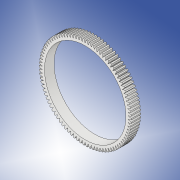
# Autodesk Inventor part: Flexspline
Saved by Autodesk Inventor 2017 (Build 210142000, 142)
## iProperties
Created: 2017-07-11
Part Number: Flexspline
Material: ABS Plastic
Document SubType Name: Modeling
Designer: zallen
Density: 1.06 g/cm^3
Appearance: CR White
Author: zallen
Autodesk Inventor part; units mm, degrees
ref_plane "YZ Plane" through (0, 0, 0) normal (1, 0, 0) x (0, 1, 0)
ref_plane "XZ Plane" through (0, 0, 0) normal (0, 1, 0) x (-1, 0, 0)
ref_plane "XY Plane" through (0, 0, 0) normal (0, 0, 1) x (1, 0, 0)
sketch "Sketch1" plane through (0, 0, 0) normal (0, 0, 1) x (1, 0, 0)
  circle A0 centre (0, 0) radius 45
  circle A1 centre (0, 0) radius 48 construction
  line L0 (0, 0) -> (52.2063, 0) construction
  arc A2 (47.9962, 0.6) -> (44.9782, 1.4) centre (42.6647, -13.4205) ccw
  arc A3 (47.9962, -0.6) -> (47.9962, 0.6) centre (28.0053, 0) ccw
  arc A4 (44.9782, -1.4) -> (47.9962, -0.6) centre (42.6647, 13.4205) ccw
  arc A5 (44.9782, -1.4) -> (44.9782, 1.4) centre (0, 0) ccw
  arc A6 (47.8375, 3.9466) -> (44.771, 4.5341) centre (43.497, -10.4117) ccw
  arc A7 (44.9663, 1.7409) -> (47.9212, 2.7495) centre (41.6246, 16.364) ccw
  arc A8 (47.9212, 2.7495) -> (47.8375, 3.9466) centre (27.937, 1.9535) ccw
  circle A9 centre (0, 0) radius 45
  arc A10 (44.9663, 1.7409) -> (44.771, 4.5341) centre (0, 0) ccw
  arc A11 (47.4456, 7.2739) -> (44.3456, 7.6461) centre (44.1173, -7.3521) ccw
  arc A12 (44.7353, 4.8734) -> (47.6127, 6.0856) centre (40.3818, 19.2277) ccw
  arc A13 (47.6127, 6.0856) -> (47.4456, 7.2739) centre (27.7327, 3.8976) ccw
  circle A14 centre (0, 0) radius 45
  arc A15 (44.7353, 4.8734) -> (44.3456, 7.6461) centre (0, 0) ccw
  arc A16 (46.8227, 10.5659) -> (43.7043, 10.7209) centre (44.5227, -4.2568) ccw
  arc A17 (44.2864, 7.9821) -> (47.0722, 9.3921) centre (38.9421, 21.9977) ccw
  arc A18 (47.0722, 9.3921) -> (46.8227, 10.5659) centre (27.3933, 5.8226) ccw
  circle A19 centre (0, 0) radius 45
  arc A20 (44.2864, 7.9821) -> (43.7043, 10.7209) centre (0, 0) ccw
  arc A21 (45.9716, 13.8063) -> (42.8499, 13.7434) centre (44.7112, -1.1406) ccw
  arc A22 (43.6217, 11.0519) -> (46.3023, 12.6528) centre (37.3128, 24.6606) ccw
  arc A23 (46.3023, 12.6528) -> (45.9716, 13.8063) centre (26.9204, 7.7193) ccw
  circle A24 centre (0, 0) radius 45
  arc A25 (43.6217, 11.0519) -> (42.8499, 13.7434) centre (0, 0) ccw
  arc A26 (44.8965, 16.9795) -> (41.7869, 16.699) centre (44.6818, 1.981) ccw
  arc A27 (42.7445, 14.0679) -> (45.3069, 15.8519) centre (35.5017, 27.2034) ccw
  arc A28 (45.3069, 15.8519) -> (44.8965, 16.9795) centre (26.3163, 9.5784) ccw
  circle A29 centre (0, 0) radius 45
  arc A30 (42.7445, 14.0679) -> (41.7869, 16.699) centre (0, 0) ccw
  arc A31 (43.6027, 20.07) -> (40.5202, 19.5733) centre (44.4348, 5.0931) ccw
  arc A32 (41.6591, 17.0153) -> (44.0908, 18.9737) centre (33.5176, 29.6136) ccw
  arc A33 (44.0908, 18.9737) -> (43.6027, 20.07) centre (25.5841, 11.3908) ccw
  circle A34 centre (0, 0) radius 45
  arc A35 (41.6591, 17.0153) -> (40.5202, 19.5733) centre (0, 0) ccw
  arc A36 (42.0965, 23.0626) -> (39.0561, 22.3521) centre (43.9713, 8.1803) ccw
  arc A37 (40.3707, 19.8799) -> (42.6599, 22.0031) centre (31.3702, 31.8795) ccw
  arc A38 (42.6599, 22.0031) -> (42.0965, 23.0626) centre (24.7272, 13.1477) ccw
  circle A39 centre (0, 0) radius 45
  arc A40 (40.3707, 19.8799) -> (39.0561, 22.3521) centre (0, 0) ccw
  arc A41 (40.3852, 25.943) -> (37.4018, 25.0221) centre (43.2935, 11.2276) ccw
  arc A42 (38.8856, 22.6476) -> (41.0211, 24.9253) centre (29.07, 33.9901) ccw
  arc A43 (41.0211, 24.9253) -> (40.3852, 25.943) centre (23.7498, 14.8405) ccw
  circle A44 centre (0, 0) radius 45
  arc A45 (38.8856, 22.6476) -> (37.4018, 25.0221) centre (0, 0) ccw
  arc A46 (38.4771, 28.6969) -> (35.5652, 27.5702) centre (42.4049, 14.2203) ccw
  arc A47 (37.211, 25.3049) -> (39.1825, 27.7261) centre (26.6281, 35.9351) ccw
  arc A48 (39.1825, 27.7261) -> (38.4771, 28.6969) centre (22.6567, 16.4611) ccw
  circle A49 centre (0, 0) radius 45
  arc A50 (37.211, 25.3049) -> (35.5652, 27.5702) centre (0, 0) ccw
  arc A51 (36.3816, 31.311) -> (33.5554, 29.9839) centre (41.3096, 17.1437) ccw
  arc A52 (35.3552, 27.839) -> (37.1529, 30.3918) centre (24.0565, 37.7051) ccw
  arc A53 (37.1529, 30.3918) -> (36.3816, 31.311) centre (21.4533, 18.0014) ccw
  circle A54 centre (0, 0) radius 45
  arc A55 (35.3552, 27.839) -> (33.5554, 29.9839) centre (0, 0) ccw
  arc A56 (34.1088, 33.7726) -> (31.3821, 32.2516) centre (40.0131, 19.9835) ccw
  arc A57 (33.3271, 30.2374) -> (34.9424, 32.9094) centre (21.3678, 39.2913) ccw
  arc A58 (34.9424, 32.9094) -> (34.1088, 33.7726) centre (20.1453, 19.4541) ccw
  circle A59 centre (0, 0) radius 45
  arc A60 (33.3271, 30.2374) -> (31.3821, 32.2516) centre (0, 0) ccw
  arc A61 (31.6699, 36.0696) -> (29.0559, 34.3621) centre (38.5217, 22.726) ccw
  arc A62 (31.1367, 32.4885) -> (32.5616, 35.2667) centre (18.5749, 40.6862) ccw
  arc A63 (32.5616, 35.2667) -> (31.6699, 36.0696) centre (18.7392, 20.812) ccw
  circle A64 centre (0, 0) radius 45
  arc A65 (31.1367, 32.4885) -> (29.0559, 34.3621) centre (0, 0) ccw
  arc A66 (29.0766, 38.191) -> (26.5881, 36.3052) centre (36.8425, 25.3578) ccw
  arc A67 (28.7946, 34.5814) -> (30.0222, 37.4522) centre (15.6915, 41.8828) ccw
  arc A68 (30.0222, 37.4522) -> (29.0766, 38.191) centre (17.2418, 22.0684) ccw
  circle A69 centre (0, 0) radius 45
  arc A70 (28.7946, 34.5814) -> (26.5881, 36.3052) centre (0, 0) ccw
  arc A71 (26.3417, 40.1262) -> (23.9908, 38.0715) centre (34.9839, 27.866) ccw
  arc A72 (26.3122, 36.5058) -> (27.3366, 39.4552) centre (12.7317, 42.8753) ccw
  arc A73 (27.3366, 39.4552) -> (26.3417, 40.1262) centre (15.6603, 23.2174) ccw
  circle A74 centre (0, 0) radius 45
  arc A75 (26.3122, 36.5058) -> (23.9908, 38.0715) centre (0, 0) ccw
  arc A76 (23.4785, 41.866) -> (21.2767, 39.6523) centre (32.9549, 30.2385) ccw
  arc A77 (23.7015, 38.2523) -> (24.5177, 41.266) centre (9.7099, 43.659) ccw
  arc A78 (24.5177, 41.266) -> (23.4785, 41.866) centre (14.0026, 24.2533) ccw
  circle A79 centre (0, 0) radius 45
  arc A80 (23.7015, 38.2523) -> (21.2767, 39.6523) centre (0, 0) ccw
  arc A81 (20.5009, 43.4018) -> (18.4588, 41.0399) centre (30.7653, 32.4636) ccw
  arc A82 (20.9755, 39.8124) -> (21.5794, 42.8757) centre (6.6407, 44.23) ccw
  arc A83 (21.5794, 42.8757) -> (20.5009, 43.4018) centre (12.2767, 25.171) ccw
  circle A84 centre (0, 0) radius 45
  arc A85 (20.9755, 39.8124) -> (18.4588, 41.0399) centre (0, 0) ccw
  arc A86 (17.4234, 44.7261) -> (15.5511, 42.2275) centre (28.4258, 34.5306) ccw
  arc A87 (18.1472, 41.1786) -> (18.536, 44.2766) centre (3.5392, 44.5855) ccw
  arc A88 (18.536, 44.2766) -> (17.4234, 44.7261) centre (10.491, 25.966) ccw
  circle A89 centre (0, 0) radius 45
  arc A90 (18.1472, 41.1786) -> (15.5511, 42.2275) centre (0, 0) ccw
  arc A91 (14.261, 45.8326) -> (12.5676, 43.2095) centre (25.9478, 36.4294) ccw
  arc A92 (15.2305, 42.3442) -> (15.4023, 45.4617) centre (0.4205, 44.7237) ccw
  arc A93 (15.4023, 45.4617) -> (14.261, 45.8326) centre (8.6541, 26.6346) ccw
  circle A94 centre (0, 0) radius 45
  arc A95 (15.2305, 42.3442) -> (12.5676, 43.2095) centre (0, 0) ccw
  arc A96 (11.0292, 46.7157) -> (9.5228, 43.9809) centre (23.3434, 38.1507) ccw
  arc A97 (12.2396, 43.3035) -> (12.1935, 46.4254) centre (-2.7003, 44.6441) ccw
  arc A98 (12.1935, 46.4254) -> (11.0292, 46.7157) centre (6.7751, 27.1734) ccw
  circle A99 centre (0, 0) radius 45
  arc A100 (12.2396, 43.3035) -> (9.5228, 43.9809) centre (0, 0) ccw
  arc A101 (7.7436, 47.3713) -> (6.4317, 44.538) centre (20.6253, 39.6861) ccw
  arc A102 (9.1891, 44.0518) -> (8.9253, 47.1629) centre (-5.808, 44.347) ccw
  arc A103 (8.9253, 47.1629) -> (7.7436, 47.3713) centre (4.8631, 27.5798) ccw
  circle A104 centre (0, 0) radius 45
  arc A105 (9.1891, 44.0518) -> (6.4317, 44.538) centre (0, 0) ccw
  arc A106 (4.4203, 47.796) -> (3.3092, 44.8782) centre (17.8067, 41.0282) ccw
  arc A107 (6.0938, 44.5855) -> (5.6137, 47.6706) centre (-8.8873, 43.8338) ccw
  arc A108 (5.6137, 47.6706) -> (4.4203, 47.796) centre (2.9273, 27.8518) ccw
  circle A109 centre (0, 0) radius 45
  arc A110 (6.0938, 44.5855) -> (3.3092, 44.8782) centre (0, 0) ccw
  arc A111 (1.0754, 47.988) -> (0.1706, 44.9997) centre (14.9013, 42.1704) ccw
  arc A112 (2.9689, 44.902) -> (2.2747, 47.9461) centre (-11.9234, 43.1071) ccw
  arc A113 (2.2747, 47.9461) -> (1.0754, 47.988) centre (0.9774, 27.9882) ccw
  circle A114 centre (0, 0) radius 45
  arc A115 (2.9689, 44.902) -> (0.1706, 44.9997) centre (0, 0) ccw
  arc A116 (-2.2747, 47.9461) -> (-2.9689, 44.902) centre (11.9234, 43.1071) ccw
  arc A117 (-0.1706, 44.9997) -> (-1.0754, 47.988) centre (-14.9013, 42.1704) ccw
  arc A118 (-1.0754, 47.988) -> (-2.2747, 47.9461) centre (-0.9774, 27.9882) ccw
  circle A119 centre (0, 0) radius 45
  arc A120 (-0.1706, 44.9997) -> (-2.9689, 44.902) centre (0, 0) ccw
  arc A121 (-5.6137, 47.6706) -> (-6.0938, 44.5855) centre (8.8873, 43.8338) ccw
  arc A122 (-3.3092, 44.8782) -> (-4.4203, 47.796) centre (-17.8067, 41.0282) ccw
  arc A123 (-4.4203, 47.796) -> (-5.6137, 47.6706) centre (-2.9273, 27.8518) ccw
  circle A124 centre (0, 0) radius 45
  arc A125 (-3.3092, 44.8782) -> (-6.0938, 44.5855) centre (0, 0) ccw
  arc A126 (-8.9253, 47.1629) -> (-9.1891, 44.0518) centre (5.808, 44.347) ccw
  arc A127 (-6.4317, 44.538) -> (-7.7436, 47.3713) centre (-20.6253, 39.6861) ccw
  arc A128 (-7.7436, 47.3713) -> (-8.9253, 47.1629) centre (-4.8631, 27.5798) ccw
  circle A129 centre (0, 0) radius 45
  arc A130 (-6.4317, 44.538) -> (-9.1891, 44.0518) centre (0, 0) ccw
  arc A131 (-12.1935, 46.4254) -> (-12.2396, 43.3035) centre (2.7003, 44.6441) ccw
  arc A132 (-9.5228, 43.9809) -> (-11.0292, 46.7157) centre (-23.3434, 38.1507) ccw
  arc A133 (-11.0292, 46.7157) -> (-12.1935, 46.4254) centre (-6.7751, 27.1734) ccw
  circle A134 centre (0, 0) radius 45
  arc A135 (-9.5228, 43.9809) -> (-12.2396, 43.3035) centre (0, 0) ccw
  arc A136 (-15.4023, 45.4617) -> (-15.2305, 42.3442) centre (-0.4205, 44.7237) ccw
  arc A137 (-12.5676, 43.2095) -> (-14.261, 45.8326) centre (-25.9478, 36.4294) ccw
  arc A138 (-14.261, 45.8326) -> (-15.4023, 45.4617) centre (-8.6541, 26.6346) ccw
  circle A139 centre (0, 0) radius 45
  arc A140 (-12.5676, 43.2095) -> (-15.2305, 42.3442) centre (0, 0) ccw
  arc A141 (-18.536, 44.2766) -> (-18.1472, 41.1786) centre (-3.5392, 44.5855) ccw
  arc A142 (-15.5511, 42.2275) -> (-17.4234, 44.7261) centre (-28.4258, 34.5306) ccw
  arc A143 (-17.4234, 44.7261) -> (-18.536, 44.2766) centre (-10.491, 25.966) ccw
  circle A144 centre (0, 0) radius 45
  arc A145 (-15.5511, 42.2275) -> (-18.1472, 41.1786) centre (0, 0) ccw
  arc A146 (-21.5794, 42.8757) -> (-20.9755, 39.8124) centre (-6.6407, 44.23) ccw
  arc A147 (-18.4588, 41.0399) -> (-20.5009, 43.4018) centre (-30.7653, 32.4636) ccw
  arc A148 (-20.5009, 43.4018) -> (-21.5794, 42.8757) centre (-12.2767, 25.171) ccw
  circle A149 centre (0, 0) radius 45
  arc A150 (-18.4588, 41.0399) -> (-20.9755, 39.8124) centre (0, 0) ccw
  arc A151 (-24.5177, 41.266) -> (-23.7015, 38.2523) centre (-9.7099, 43.659) ccw
  arc A152 (-21.2767, 39.6523) -> (-23.4785, 41.866) centre (-32.9549, 30.2385) ccw
  arc A153 (-23.4785, 41.866) -> (-24.5177, 41.266) centre (-14.0026, 24.2533) ccw
  circle A154 centre (0, 0) radius 45
  arc A155 (-21.2767, 39.6523) -> (-23.7015, 38.2523) centre (0, 0) ccw
  arc A156 (-27.3366, 39.4552) -> (-26.3122, 36.5058) centre (-12.7317, 42.8753) ccw
  arc A157 (-23.9908, 38.0715) -> (-26.3417, 40.1262) centre (-34.9839, 27.866) ccw
  arc A158 (-26.3417, 40.1262) -> (-27.3366, 39.4552) centre (-15.6603, 23.2174) ccw
  circle A159 centre (0, 0) radius 45
  arc A160 (-23.9908, 38.0715) -> (-26.3122, 36.5058) centre (0, 0) ccw
  arc A161 (-30.0222, 37.4522) -> (-28.7946, 34.5814) centre (-15.6915, 41.8828) ccw
  arc A162 (-26.5881, 36.3052) -> (-29.0766, 38.191) centre (-36.8425, 25.3578) ccw
  arc A163 (-29.0766, 38.191) -> (-30.0222, 37.4522) centre (-17.2418, 22.0684) ccw
  circle A164 centre (0, 0) radius 45
  arc A165 (-26.5881, 36.3052) -> (-28.7946, 34.5814) centre (0, 0) ccw
  arc A166 (-32.5616, 35.2667) -> (-31.1367, 32.4885) centre (-18.5749, 40.6862) ccw
  arc A167 (-29.0559, 34.3621) -> (-31.6699, 36.0696) centre (-38.5217, 22.726) ccw
  arc A168 (-31.6699, 36.0696) -> (-32.5616, 35.2667) centre (-18.7392, 20.812) ccw
  circle A169 centre (0, 0) radius 45
  arc A170 (-29.0559, 34.3621) -> (-31.1367, 32.4885) centre (0, 0) ccw
  arc A171 (-34.9424, 32.9094) -> (-33.3271, 30.2374) centre (-21.3678, 39.2913) ccw
  arc A172 (-31.3821, 32.2516) -> (-34.1088, 33.7726) centre (-40.0131, 19.9835) ccw
  arc A173 (-34.1088, 33.7726) -> (-34.9424, 32.9094) centre (-20.1453, 19.4541) ccw
  circle A174 centre (0, 0) radius 45
  arc A175 (-31.3821, 32.2516) -> (-33.3271, 30.2374) centre (0, 0) ccw
  arc A176 (-37.1529, 30.3918) -> (-35.3552, 27.839) centre (-24.0565, 37.7051) ccw
  arc A177 (-33.5554, 29.9839) -> (-36.3816, 31.311) centre (-41.3096, 17.1437) ccw
  arc A178 (-36.3816, 31.311) -> (-37.1529, 30.3918) centre (-21.4533, 18.0014) ccw
  circle A179 centre (0, 0) radius 45
  arc A180 (-33.5554, 29.9839) -> (-35.3552, 27.839) centre (0, 0) ccw
  arc A181 (-39.1825, 27.7261) -> (-37.211, 25.3049) centre (-26.6281, 35.9351) ccw
  arc A182 (-35.5652, 27.5702) -> (-38.4771, 28.6969) centre (-42.4049, 14.2203) ccw
  arc A183 (-38.4771, 28.6969) -> (-39.1825, 27.7261) centre (-22.6567, 16.4611) ccw
  circle A184 centre (0, 0) radius 45
  arc A185 (-35.5652, 27.5702) -> (-37.211, 25.3049) centre (0, 0) ccw
  arc A186 (-41.0211, 24.9253) -> (-38.8856, 22.6476) centre (-29.07, 33.9901) ccw
  arc A187 (-37.4018, 25.0221) -> (-40.3852, 25.943) centre (-43.2935, 11.2276) ccw
  arc A188 (-40.3852, 25.943) -> (-41.0211, 24.9253) centre (-23.7498, 14.8405) ccw
  circle A189 centre (0, 0) radius 45
  arc A190 (-37.4018, 25.0221) -> (-38.8856, 22.6476) centre (0, 0) ccw
  arc A191 (-42.6599, 22.0031) -> (-40.3707, 19.8799) centre (-31.3702, 31.8795) ccw
  arc A192 (-39.0561, 22.3521) -> (-42.0965, 23.0626) centre (-43.9713, 8.1803) ccw
  arc A193 (-42.0965, 23.0626) -> (-42.6599, 22.0031) centre (-24.7272, 13.1477) ccw
  circle A194 centre (0, 0) radius 45
  arc A195 (-39.0561, 22.3521) -> (-40.3707, 19.8799) centre (0, 0) ccw
  arc A196 (-44.0908, 18.9737) -> (-41.6591, 17.0153) centre (-33.5176, 29.6136) ccw
  arc A197 (-40.5202, 19.5733) -> (-43.6027, 20.07) centre (-44.4348, 5.0931) ccw
  arc A198 (-43.6027, 20.07) -> (-44.0908, 18.9737) centre (-25.5841, 11.3908) ccw
  circle A199 centre (0, 0) radius 45
  arc A200 (-40.5202, 19.5733) -> (-41.6591, 17.0153) centre (0, 0) ccw
  arc A201 (-45.3069, 15.8519) -> (-42.7445, 14.0679) centre (-35.5017, 27.2034) ccw
  arc A202 (-41.7869, 16.699) -> (-44.8965, 16.9795) centre (-44.6818, 1.981) ccw
  arc A203 (-44.8965, 16.9795) -> (-45.3069, 15.8519) centre (-26.3163, 9.5784) ccw
  circle A204 centre (0, 0) radius 45
  arc A205 (-41.7869, 16.699) -> (-42.7445, 14.0679) centre (0, 0) ccw
  arc A206 (-46.3023, 12.6528) -> (-43.6217, 11.0519) centre (-37.3128, 24.6606) ccw
  arc A207 (-42.8499, 13.7434) -> (-45.9716, 13.8063) centre (-44.7112, -1.1406) ccw
  arc A208 (-45.9716, 13.8063) -> (-46.3023, 12.6528) centre (-26.9204, 7.7193) ccw
  circle A209 centre (0, 0) radius 45
  arc A210 (-42.8499, 13.7434) -> (-43.6217, 11.0519) centre (0, 0) ccw
  arc A211 (-47.0722, 9.3921) -> (-44.2864, 7.9821) centre (-38.9421, 21.9977) ccw
  arc A212 (-43.7043, 10.7209) -> (-46.8227, 10.5659) centre (-44.5227, -4.2568) ccw
  arc A213 (-46.8227, 10.5659) -> (-47.0722, 9.3921) centre (-27.3933, 5.8226) ccw
  circle A214 centre (0, 0) radius 45
  arc A215 (-43.7043, 10.7209) -> (-44.2864, 7.9821) centre (0, 0) ccw
  arc A216 (-47.6127, 6.0856) -> (-44.7353, 4.8734) centre (-40.3818, 19.2277) ccw
  arc A217 (-44.3456, 7.6461) -> (-47.4456, 7.2739) centre (-44.1173, -7.3521) ccw
  arc A218 (-47.4456, 7.2739) -> (-47.6127, 6.0856) centre (-27.7327, 3.8976) ccw
  circle A219 centre (0, 0) radius 45
  arc A220 (-44.3456, 7.6461) -> (-44.7353, 4.8734) centre (0, 0) ccw
  arc A221 (-47.9212, 2.7495) -> (-44.9663, 1.7409) centre (-41.6246, 16.364) ccw
  arc A222 (-44.771, 4.5341) -> (-47.8375, 3.9466) centre (-43.497, -10.4117) ccw
  arc A223 (-47.8375, 3.9466) -> (-47.9212, 2.7495) centre (-27.937, 1.9535) ccw
  circle A224 centre (0, 0) radius 45
  arc A225 (-44.771, 4.5341) -> (-44.9663, 1.7409) centre (0, 0) ccw
  arc A226 (-47.9962, -0.6) -> (-44.9782, -1.4) centre (-42.6647, 13.4205) ccw
  arc A227 (-44.9782, 1.4) -> (-47.9962, 0.6) centre (-42.6647, -13.4205) ccw
  arc A228 (-47.9962, 0.6) -> (-47.9962, -0.6) centre (-28.0053, 0) ccw
  circle A229 centre (0, 0) radius 45
  arc A230 (-44.9782, 1.4) -> (-44.9782, -1.4) centre (0, 0) ccw
  arc A231 (-47.8375, -3.9466) -> (-44.771, -4.5341) centre (-43.497, 10.4117) ccw
  arc A232 (-44.9663, -1.7409) -> (-47.9212, -2.7495) centre (-41.6246, -16.364) ccw
  arc A233 (-47.9212, -2.7495) -> (-47.8375, -3.9466) centre (-27.937, -1.9535) ccw
  circle A234 centre (0, 0) radius 45
  arc A235 (-44.9663, -1.7409) -> (-44.771, -4.5341) centre (0, 0) ccw
  arc A236 (-47.4456, -7.2739) -> (-44.3456, -7.6461) centre (-44.1173, 7.3521) ccw
  arc A237 (-44.7353, -4.8734) -> (-47.6127, -6.0856) centre (-40.3818, -19.2277) ccw
  arc A238 (-47.6127, -6.0856) -> (-47.4456, -7.2739) centre (-27.7327, -3.8976) ccw
  circle A239 centre (0, 0) radius 45
  arc A240 (-44.7353, -4.8734) -> (-44.3456, -7.6461) centre (0, 0) ccw
  arc A241 (-46.8227, -10.5659) -> (-43.7043, -10.7209) centre (-44.5227, 4.2568) ccw
  arc A242 (-44.2864, -7.9821) -> (-47.0722, -9.3921) centre (-38.9421, -21.9977) ccw
  arc A243 (-47.0722, -9.3921) -> (-46.8227, -10.5659) centre (-27.3933, -5.8226) ccw
  circle A244 centre (0, 0) radius 45
  arc A245 (-44.2864, -7.9821) -> (-43.7043, -10.7209) centre (0, 0) ccw
  arc A246 (-45.9716, -13.8063) -> (-42.8499, -13.7434) centre (-44.7112, 1.1406) ccw
  arc A247 (-43.6217, -11.0519) -> (-46.3023, -12.6528) centre (-37.3128, -24.6606) ccw
  arc A248 (-46.3023, -12.6528) -> (-45.9716, -13.8063) centre (-26.9204, -7.7193) ccw
  circle A249 centre (0, 0) radius 45
  arc A250 (-43.6217, -11.0519) -> (-42.8499, -13.7434) centre (0, 0) ccw
  arc A251 (-44.8965, -16.9795) -> (-41.7869, -16.699) centre (-44.6818, -1.981) ccw
  arc A252 (-42.7445, -14.0679) -> (-45.3069, -15.8519) centre (-35.5017, -27.2034) ccw
  arc A253 (-45.3069, -15.8519) -> (-44.8965, -16.9795) centre (-26.3163, -9.5784) ccw
  circle A254 centre (0, 0) radius 45
  arc A255 (-42.7445, -14.0679) -> (-41.7869, -16.699) centre (0, 0) ccw
  arc A256 (-43.6027, -20.07) -> (-40.5202, -19.5733) centre (-44.4348, -5.0931) ccw
  arc A257 (-41.6591, -17.0153) -> (-44.0908, -18.9737) centre (-33.5176, -29.6136) ccw
  arc A258 (-44.0908, -18.9737) -> (-43.6027, -20.07) centre (-25.5841, -11.3908) ccw
  circle A259 centre (0, 0) radius 45
  arc A260 (-41.6591, -17.0153) -> (-40.5202, -19.5733) centre (0, 0) ccw
  arc A261 (-42.0965, -23.0626) -> (-39.0561, -22.3521) centre (-43.9713, -8.1803) ccw
  arc A262 (-40.3707, -19.8799) -> (-42.6599, -22.0031) centre (-31.3702, -31.8795) ccw
  arc A263 (-42.6599, -22.0031) -> (-42.0965, -23.0626) centre (-24.7272, -13.1477) ccw
  circle A264 centre (0, 0) radius 45
  arc A265 (-40.3707, -19.8799) -> (-39.0561, -22.3521) centre (0, 0) ccw
  arc A266 (-40.3852, -25.943) -> (-37.4018, -25.0221) centre (-43.2935, -11.2276) ccw
  arc A267 (-38.8856, -22.6476) -> (-41.0211, -24.9253) centre (-29.07, -33.9901) ccw
  arc A268 (-41.0211, -24.9253) -> (-40.3852, -25.943) centre (-23.7498, -14.8405) ccw
  circle A269 centre (0, 0) radius 45
  arc A270 (-38.8856, -22.6476) -> (-37.4018, -25.0221) centre (0, 0) ccw
  arc A271 (-38.4771, -28.6969) -> (-35.5652, -27.5702) centre (-42.4049, -14.2203) ccw
  arc A272 (-37.211, -25.3049) -> (-39.1825, -27.7261) centre (-26.6281, -35.9351) ccw
  arc A273 (-39.1825, -27.7261) -> (-38.4771, -28.6969) centre (-22.6567, -16.4611) ccw
  circle A274 centre (0, 0) radius 45
  arc A275 (-37.211, -25.3049) -> (-35.5652, -27.5702) centre (0, 0) ccw
  arc A276 (-36.3816, -31.311) -> (-33.5554, -29.9839) centre (-41.3096, -17.1437) ccw
  arc A277 (-35.3552, -27.839) -> (-37.1529, -30.3918) centre (-24.0565, -37.7051) ccw
  arc A278 (-37.1529, -30.3918) -> (-36.3816, -31.311) centre (-21.4533, -18.0014) ccw
  circle A279 centre (0, 0) radius 45
  arc A280 (-35.3552, -27.839) -> (-33.5554, -29.9839) centre (0, 0) ccw
  arc A281 (-34.1088, -33.7726) -> (-31.3821, -32.2516) centre (-40.0131, -19.9835) ccw
  arc A282 (-33.3271, -30.2374) -> (-34.9424, -32.9094) centre (-21.3678, -39.2913) ccw
  arc A283 (-34.9424, -32.9094) -> (-34.1088, -33.7726) centre (-20.1453, -19.4541) ccw
  circle A284 centre (0, 0) radius 45
  arc A285 (-33.3271, -30.2374) -> (-31.3821, -32.2516) centre (0, 0) ccw
  arc A286 (-31.6699, -36.0696) -> (-29.0559, -34.3621) centre (-38.5217, -22.726) ccw
  arc A287 (-31.1367, -32.4885) -> (-32.5616, -35.2667) centre (-18.5749, -40.6862) ccw
  arc A288 (-32.5616, -35.2667) -> (-31.6699, -36.0696) centre (-18.7392, -20.812) ccw
  circle A289 centre (0, 0) radius 45
  arc A290 (-31.1367, -32.4885) -> (-29.0559, -34.3621) centre (0, 0) ccw
  arc A291 (-29.0766, -38.191) -> (-26.5881, -36.3052) centre (-36.8425, -25.3578) ccw
  arc A292 (-28.7946, -34.5814) -> (-30.0222, -37.4522) centre (-15.6915, -41.8828) ccw
  arc A293 (-30.0222, -37.4522) -> (-29.0766, -38.191) centre (-17.2418, -22.0684) ccw
  circle A294 centre (0, 0) radius 45
  arc A295 (-28.7946, -34.5814) -> (-26.5881, -36.3052) centre (0, 0) ccw
  arc A296 (-26.3417, -40.1262) -> (-23.9908, -38.0715) centre (-34.9839, -27.866) ccw
  arc A297 (-26.3122, -36.5058) -> (-27.3366, -39.4552) centre (-12.7317, -42.8753) ccw
  arc A298 (-27.3366, -39.4552) -> (-26.3417, -40.1262) centre (-15.6603, -23.2174) ccw
  circle A299 centre (0, 0) radius 45
  arc A300 (-26.3122, -36.5058) -> (-23.9908, -38.0715) centre (0, 0) ccw
  arc A301 (-23.4785, -41.866) -> (-21.2767, -39.6523) centre (-32.9549, -30.2385) ccw
  arc A302 (-23.7015, -38.2523) -> (-24.5177, -41.266) centre (-9.7099, -43.659) ccw
  arc A303 (-24.5177, -41.266) -> (-23.4785, -41.866) centre (-14.0026, -24.2533) ccw
  circle A304 centre (0, 0) radius 45
  arc A305 (-23.7015, -38.2523) -> (-21.2767, -39.6523) centre (0, 0) ccw
  arc A306 (-20.5009, -43.4018) -> (-18.4588, -41.0399) centre (-30.7653, -32.4636) ccw
  arc A307 (-20.9755, -39.8124) -> (-21.5794, -42.8757) centre (-6.6407, -44.23) ccw
  arc A308 (-21.5794, -42.8757) -> (-20.5009, -43.4018) centre (-12.2767, -25.171) ccw
  circle A309 centre (0, 0) radius 45
  arc A310 (-20.9755, -39.8124) -> (-18.4588, -41.0399) centre (0, 0) ccw
  arc A311 (-17.4234, -44.7261) -> (-15.5511, -42.2275) centre (-28.4258, -34.5306) ccw
  arc A312 (-18.1472, -41.1786) -> (-18.536, -44.2766) centre (-3.5392, -44.5855) ccw
  arc A313 (-18.536, -44.2766) -> (-17.4234, -44.7261) centre (-10.491, -25.966) ccw
  circle A314 centre (0, 0) radius 45
  arc A315 (-18.1472, -41.1786) -> (-15.5511, -42.2275) centre (0, 0) ccw
  arc A316 (-14.261, -45.8326) -> (-12.5676, -43.2095) centre (-25.9478, -36.4294) ccw
  arc A317 (-15.2305, -42.3442) -> (-15.4023, -45.4617) centre (-0.4205, -44.7237) ccw
  arc A318 (-15.4023, -45.4617) -> (-14.261, -45.8326) centre (-8.6541, -26.6346) ccw
  circle A319 centre (0, 0) radius 45
  arc A320 (-15.2305, -42.3442) -> (-12.5676, -43.2095) centre (0, 0) ccw
  arc A321 (-11.0292, -46.7157) -> (-9.5228, -43.9809) centre (-23.3434, -38.1507) ccw
  arc A322 (-12.2396, -43.3035) -> (-12.1935, -46.4254) centre (2.7003, -44.6441) ccw
  arc A323 (-12.1935, -46.4254) -> (-11.0292, -46.7157) centre (-6.7751, -27.1734) ccw
  circle A324 centre (0, 0) radius 45
  arc A325 (-12.2396, -43.3035) -> (-9.5228, -43.9809) centre (0, 0) ccw
  arc A326 (-7.7436, -47.3713) -> (-6.4317, -44.538) centre (-20.6253, -39.6861) ccw
  arc A327 (-9.1891, -44.0518) -> (-8.9253, -47.1629) centre (5.808, -44.347) ccw
  arc A328 (-8.9253, -47.1629) -> (-7.7436, -47.3713) centre (-4.8631, -27.5798) ccw
  circle A329 centre (0, 0) radius 45
  arc A330 (-9.1891, -44.0518) -> (-6.4317, -44.538) centre (0, 0) ccw
  arc A331 (-4.4203, -47.796) -> (-3.3092, -44.8782) centre (-17.8067, -41.0282) ccw
  arc A332 (-6.0938, -44.5855) -> (-5.6137, -47.6706) centre (8.8873, -43.8338) ccw
  arc A333 (-5.6137, -47.6706) -> (-4.4203, -47.796) centre (-2.9273, -27.8518) ccw
  circle A334 centre (0, 0) radius 45
  arc A335 (-6.0938, -44.5855) -> (-3.3092, -44.8782) centre (0, 0) ccw
  arc A336 (-1.0754, -47.988) -> (-0.1706, -44.9997) centre (-14.9013, -42.1704) ccw
  arc A337 (-2.9689, -44.902) -> (-2.2747, -47.9461) centre (11.9234, -43.1071) ccw
  arc A338 (-2.2747, -47.9461) -> (-1.0754, -47.988) centre (-0.9774, -27.9882) ccw
  circle A339 centre (0, 0) radius 45
  arc A340 (-2.9689, -44.902) -> (-0.1706, -44.9997) centre (0, 0) ccw
  arc A341 (2.2747, -47.9461) -> (2.9689, -44.902) centre (-11.9234, -43.1071) ccw
  arc A342 (0.1706, -44.9997) -> (1.0754, -47.988) centre (14.9013, -42.1704) ccw
  arc A343 (1.0754, -47.988) -> (2.2747, -47.9461) centre (0.9774, -27.9882) ccw
  circle A344 centre (0, 0) radius 45
  arc A345 (0.1706, -44.9997) -> (2.9689, -44.902) centre (0, 0) ccw
  arc A346 (5.6137, -47.6706) -> (6.0938, -44.5855) centre (-8.8873, -43.8338) ccw
  arc A347 (3.3092, -44.8782) -> (4.4203, -47.796) centre (17.8067, -41.0282) ccw
  arc A348 (4.4203, -47.796) -> (5.6137, -47.6706) centre (2.9273, -27.8518) ccw
  circle A349 centre (0, 0) radius 45
  arc A350 (3.3092, -44.8782) -> (6.0938, -44.5855) centre (0, 0) ccw
  arc A351 (8.9253, -47.1629) -> (9.1891, -44.0518) centre (-5.808, -44.347) ccw
  arc A352 (6.4317, -44.538) -> (7.7436, -47.3713) centre (20.6253, -39.6861) ccw
  arc A353 (7.7436, -47.3713) -> (8.9253, -47.1629) centre (4.8631, -27.5798) ccw
  circle A354 centre (0, 0) radius 45
  arc A355 (6.4317, -44.538) -> (9.1891, -44.0518) centre (0, 0) ccw
  arc A356 (12.1935, -46.4254) -> (12.2396, -43.3035) centre (-2.7003, -44.6441) ccw
  arc A357 (9.5228, -43.9809) -> (11.0292, -46.7157) centre (23.3434, -38.1507) ccw
  arc A358 (11.0292, -46.7157) -> (12.1935, -46.4254) centre (6.7751, -27.1734) ccw
  circle A359 centre (0, 0) radius 45
  arc A360 (9.5228, -43.9809) -> (12.2396, -43.3035) centre (0, 0) ccw
  arc A361 (15.4023, -45.4617) -> (15.2305, -42.3442) centre (0.4205, -44.7237) ccw
  arc A362 (12.5676, -43.2095) -> (14.261, -45.8326) centre (25.9478, -36.4294) ccw
  arc A363 (14.261, -45.8326) -> (15.4023, -45.4617) centre (8.6541, -26.6346) ccw
  circle A364 centre (0, 0) radius 45
  arc A365 (12.5676, -43.2095) -> (15.2305, -42.3442) centre (0, 0) ccw
  arc A366 (18.536, -44.2766) -> (18.1472, -41.1786) centre (3.5392, -44.5855) ccw
  arc A367 (15.5511, -42.2275) -> (17.4234, -44.7261) centre (28.4258, -34.5306) ccw
  arc A368 (17.4234, -44.7261) -> (18.536, -44.2766) centre (10.491, -25.966) ccw
  circle A369 centre (0, 0) radius 45
  arc A370 (15.5511, -42.2275) -> (18.1472, -41.1786) centre (0, 0) ccw
  arc A371 (21.5794, -42.8757) -> (20.9755, -39.8124) centre (6.6407, -44.23) ccw
  arc A372 (18.4588, -41.0399) -> (20.5009, -43.4018) centre (30.7653, -32.4636) ccw
  arc A373 (20.5009, -43.4018) -> (21.5794, -42.8757) centre (12.2767, -25.171) ccw
  circle A374 centre (0, 0) radius 45
  arc A375 (18.4588, -41.0399) -> (20.9755, -39.8124) centre (0, 0) ccw
  arc A376 (24.5177, -41.266) -> (23.7015, -38.2523) centre (9.7099, -43.659) ccw
  arc A377 (21.2767, -39.6523) -> (23.4785, -41.866) centre (32.9549, -30.2385) ccw
  arc A378 (23.4785, -41.866) -> (24.5177, -41.266) centre (14.0026, -24.2533) ccw
  circle A379 centre (0, 0) radius 45
  arc A380 (21.2767, -39.6523) -> (23.7015, -38.2523) centre (0, 0) ccw
  arc A381 (27.3366, -39.4552) -> (26.3122, -36.5058) centre (12.7317, -42.8753) ccw
  arc A382 (23.9908, -38.0715) -> (26.3417, -40.1262) centre (34.9839, -27.866) ccw
  arc A383 (26.3417, -40.1262) -> (27.3366, -39.4552) centre (15.6603, -23.2174) ccw
  circle A384 centre (0, 0) radius 45
  arc A385 (23.9908, -38.0715) -> (26.3122, -36.5058) centre (0, 0) ccw
  arc A386 (30.0222, -37.4522) -> (28.7946, -34.5814) centre (15.6915, -41.8828) ccw
  arc A387 (26.5881, -36.3052) -> (29.0766, -38.191) centre (36.8425, -25.3578) ccw
  arc A388 (29.0766, -38.191) -> (30.0222, -37.4522) centre (17.2418, -22.0684) ccw
  circle A389 centre (0, 0) radius 45
  arc A390 (26.5881, -36.3052) -> (28.7946, -34.5814) centre (0, 0) ccw
  arc A391 (32.5616, -35.2667) -> (31.1367, -32.4885) centre (18.5749, -40.6862) ccw
  arc A392 (29.0559, -34.3621) -> (31.6699, -36.0696) centre (38.5217, -22.726) ccw
  arc A393 (31.6699, -36.0696) -> (32.5616, -35.2667) centre (18.7392, -20.812) ccw
  circle A394 centre (0, 0) radius 45
  arc A395 (29.0559, -34.3621) -> (31.1367, -32.4885) centre (0, 0) ccw
  arc A396 (34.9424, -32.9094) -> (33.3271, -30.2374) centre (21.3678, -39.2913) ccw
  arc A397 (31.3821, -32.2516) -> (34.1088, -33.7726) centre (40.0131, -19.9835) ccw
  arc A398 (34.1088, -33.7726) -> (34.9424, -32.9094) centre (20.1453, -19.4541) ccw
  circle A399 centre (0, 0) radius 45
  arc A400 (31.3821, -32.2516) -> (33.3271, -30.2374) centre (0, 0) ccw
  arc A401 (37.1529, -30.3918) -> (35.3552, -27.839) centre (24.0565, -37.7051) ccw
  arc A402 (33.5554, -29.9839) -> (36.3816, -31.311) centre (41.3096, -17.1437) ccw
  arc A403 (36.3816, -31.311) -> (37.1529, -30.3918) centre (21.4533, -18.0014) ccw
  circle A404 centre (0, 0) radius 45
  arc A405 (33.5554, -29.9839) -> (35.3552, -27.839) centre (0, 0) ccw
  arc A406 (39.1825, -27.7261) -> (37.211, -25.3049) centre (26.6281, -35.9351) ccw
  arc A407 (35.5652, -27.5702) -> (38.4771, -28.6969) centre (42.4049, -14.2203) ccw
  arc A408 (38.4771, -28.6969) -> (39.1825, -27.7261) centre (22.6567, -16.4611) ccw
  circle A409 centre (0, 0) radius 45
  arc A410 (35.5652, -27.5702) -> (37.211, -25.3049) centre (0, 0) ccw
  arc A411 (41.0211, -24.9253) -> (38.8856, -22.6476) centre (29.07, -33.9901) ccw
  arc A412 (37.4018, -25.0221) -> (40.3852, -25.943) centre (43.2935, -11.2276) ccw
  arc A413 (40.3852, -25.943) -> (41.0211, -24.9253) centre (23.7498, -14.8405) ccw
  circle A414 centre (0, 0) radius 45
  arc A415 (37.4018, -25.0221) -> (38.8856, -22.6476) centre (0, 0) ccw
  arc A416 (42.6599, -22.0031) -> (40.3707, -19.8799) centre (31.3702, -31.8795) ccw
  arc A417 (39.0561, -22.3521) -> (42.0965, -23.0626) centre (43.9713, -8.1803) ccw
  arc A418 (42.0965, -23.0626) -> (42.6599, -22.0031) centre (24.7272, -13.1477) ccw
  circle A419 centre (0, 0) radius 45
  arc A420 (39.0561, -22.3521) -> (40.3707, -19.8799) centre (0, 0) ccw
  arc A421 (44.0908, -18.9737) -> (41.6591, -17.0153) centre (33.5176, -29.6136) ccw
  arc A422 (40.5202, -19.5733) -> (43.6027, -20.07) centre (44.4348, -5.0931) ccw
  arc A423 (43.6027, -20.07) -> (44.0908, -18.9737) centre (25.5841, -11.3908) ccw
  circle A424 centre (0, 0) radius 45
  arc A425 (40.5202, -19.5733) -> (41.6591, -17.0153) centre (0, 0) ccw
  arc A426 (45.3069, -15.8519) -> (42.7445, -14.0679) centre (35.5017, -27.2034) ccw
  arc A427 (41.7869, -16.699) -> (44.8965, -16.9795) centre (44.6818, -1.981) ccw
  arc A428 (44.8965, -16.9795) -> (45.3069, -15.8519) centre (26.3163, -9.5784) ccw
  circle A429 centre (0, 0) radius 45
  arc A430 (41.7869, -16.699) -> (42.7445, -14.0679) centre (0, 0) ccw
  arc A431 (46.3023, -12.6528) -> (43.6217, -11.0519) centre (37.3128, -24.6606) ccw
  arc A432 (42.8499, -13.7434) -> (45.9716, -13.8063) centre (44.7112, 1.1406) ccw
  arc A433 (45.9716, -13.8063) -> (46.3023, -12.6528) centre (26.9204, -7.7193) ccw
  circle A434 centre (0, 0) radius 45
  arc A435 (42.8499, -13.7434) -> (43.6217, -11.0519) centre (0, 0) ccw
  arc A436 (47.0722, -9.3921) -> (44.2864, -7.9821) centre (38.9421, -21.9977) ccw
  arc A437 (43.7043, -10.7209) -> (46.8227, -10.5659) centre (44.5227, 4.2568) ccw
  arc A438 (46.8227, -10.5659) -> (47.0722, -9.3921) centre (27.3933, -5.8226) ccw
  circle A439 centre (0, 0) radius 45
  arc A440 (43.7043, -10.7209) -> (44.2864, -7.9821) centre (0, 0) ccw
  arc A441 (47.6127, -6.0856) -> (44.7353, -4.8734) centre (40.3818, -19.2277) ccw
  arc A442 (44.3456, -7.6461) -> (47.4456, -7.2739) centre (44.1173, 7.3521) ccw
  arc A443 (47.4456, -7.2739) -> (47.6127, -6.0856) centre (27.7327, -3.8976) ccw
  circle A444 centre (0, 0) radius 45
  arc A445 (44.3456, -7.6461) -> (44.7353, -4.8734) centre (0, 0) ccw
  arc A446 (47.9212, -2.7495) -> (44.9663, -1.7409) centre (41.6246, -16.364) ccw
  arc A447 (44.771, -4.5341) -> (47.8375, -3.9466) centre (43.497, 10.4117) ccw
  arc A448 (47.8375, -3.9466) -> (47.9212, -2.7495) centre (27.937, -1.9535) ccw
  circle A449 centre (0, 0) radius 45
  arc A450 (44.771, -4.5341) -> (44.9663, -1.7409) centre (0, 0) ccw
  point P0 (48.0053, 0)
  point P1 (47.8883, 3.3487)
  point P2 (47.5381, 6.681)
  point P3 (46.9562, 9.9809)
  point P4 (46.1456, 13.232)
  point P5 (45.1102, 16.4188)
  point P6 (43.855, 19.5255)
  point P7 (42.3861, 22.5371)
  point P8 (40.7108, 25.4389)
  point P9 (38.8371, 28.2168)
  point P10 (36.7742, 30.8572)
  point P11 (34.5321, 33.3473)
  point P12 (32.1218, 35.6749)
  point P13 (29.555, 37.8287)
  point P14 (26.8442, 39.7982)
  point P15 (24.0026, 41.5738)
  point P16 (21.0441, 43.1468)
  point P17 (17.9831, 44.5097)
  point P18 (14.8344, 45.6557)
  point P19 (11.6135, 46.5793)
  point P20 (8.336, 47.2759)
  point P21 (5.0179, 47.7423)
  point P22 (1.6754, 47.976)
  point P23 (-1.6754, 47.976)
  point P24 (-5.0179, 47.7423)
  point P25 (-8.336, 47.2759)
  point P26 (-11.6135, 46.5793)
  point P27 (-14.8344, 45.6557)
  point P28 (-17.9831, 44.5097)
  point P29 (-21.0441, 43.1468)
  point P30 (-24.0026, 41.5738)
  point P31 (-26.8442, 39.7982)
  point P32 (-29.555, 37.8287)
  point P33 (-32.1218, 35.6749)
  point P34 (-34.5321, 33.3473)
  point P35 (-36.7742, 30.8572)
  point P36 (-38.8371, 28.2168)
  point P37 (-40.7108, 25.4389)
  point P38 (-42.3861, 22.5371)
  point P39 (-43.855, 19.5255)
  point P40 (-45.1102, 16.4188)
  point P41 (-46.1456, 13.232)
  point P42 (-46.9562, 9.9809)
  point P43 (-47.5381, 6.681)
  point P44 (-47.8883, 3.3487)
  point P45 (-48.0053, 0)
  point P46 (-47.8883, -3.3487)
  point P47 (-47.5381, -6.681)
  point P48 (-46.9562, -9.9809)
  point P49 (-46.1456, -13.232)
  point P50 (-45.1102, -16.4188)
  point P51 (-43.855, -19.5255)
  point P52 (-42.3861, -22.5371)
  point P53 (-40.7108, -25.4389)
  point P54 (-38.8371, -28.2168)
  point P55 (-36.7742, -30.8572)
  point P56 (-34.5321, -33.3473)
  point P57 (-32.1218, -35.6749)
  point P58 (-29.555, -37.8287)
  point P59 (-26.8442, -39.7982)
  point P60 (-24.0026, -41.5738)
  point P61 (-21.0441, -43.1468)
  point P62 (-17.9831, -44.5097)
  point P63 (-14.8344, -45.6557)
  point P64 (-11.6135, -46.5793)
  point P65 (-8.336, -47.2759)
  point P66 (-5.0179, -47.7423)
  point P67 (-1.6754, -47.976)
  point P68 (1.6754, -47.976)
  point P69 (5.0179, -47.7423)
  point P70 (8.336, -47.2759)
  point P71 (11.6135, -46.5793)
  point P72 (14.8344, -45.6557)
  point P73 (17.9831, -44.5097)
  point P74 (21.0441, -43.1468)
  point P75 (24.0026, -41.5738)
  point P76 (26.8442, -39.7982)
  point P77 (29.555, -37.8287)
  point P78 (32.1218, -35.6749)
  point P79 (34.5321, -33.3473)
  point P80 (36.7742, -30.8572)
  point P81 (38.8371, -28.2168)
  point P82 (40.7108, -25.4389)
  point P83 (42.3861, -22.5371)
  point P84 (43.855, -19.5255)
  point P85 (45.1102, -16.4188)
  point P86 (46.1456, -13.232)
  point P87 (46.9562, -9.9809)
  point P88 (47.5381, -6.681)
  point P89 (47.8883, -3.3487)
  dimension "d2" = 15
  dimension "d3" = 20
  dimension "d4" = 1.2
  dimension "d5" = 1.4
  dimension "d6" = 3
  dimension "d9" = 360
  constraints: 723 point on circle, 361 centre point, 2 coincident, 2 end point, 2 symmetric about line, 1 horizontal, 1 point on line, 1712 other
  measures "d2" radius of A2
  measures "d3" radius of A3
  measures "d4" distance of A1.end A1.start
  measures "d5" distance from line of L0 A2.end
extrude "Extrusion1" add sketch "Sketch1" along normal blind 10
sketch "Sketch2" plane through (0, 0, 10) normal (0, 0, 1) x (1, 0, 0)
  circle A0 centre (0, 0) radius 42.5
  dimension "d13" = 85
  constraints: 1 centre point, 1 coincident
  measures "d13" diameter of A0
extrude "Extrusion2" cut sketch "Sketch2" against normal through all
body "Solid1"
